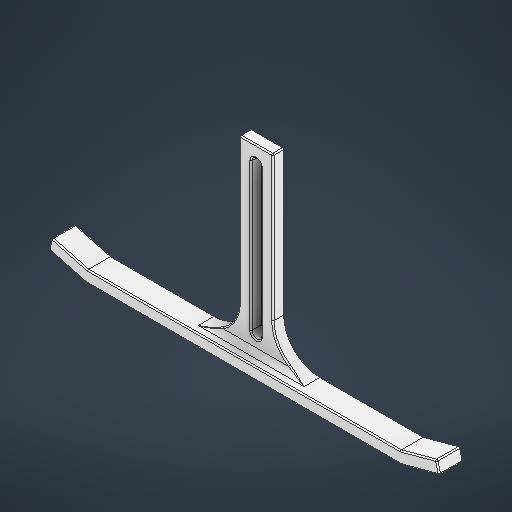
# Autodesk Inventor part: BandeV2Joint3_HALF
Saved by Autodesk Inventor 2026.2 (Build 302298010, 298A)
## iProperties
Created: 2026-06-25
Part Number: BandeV2Joint3_HALF
Material: PET Plastic
Document SubType Name: Modeling
Designer: frede
Density: 1.541 g/cm^3
Appearance: White
Author: frede
Autodesk Inventor part; units mm, degrees
ref_plane "YZ Plane" through (0, 0, 0) normal (1, 0, 0) x (0, 1, 0)
ref_plane "XZ Plane" through (0, 0, 0) normal (0, 1, 0) x (-1, 0, 0)
ref_plane "XY Plane" through (0, 0, 0) normal (0, 0, 1) x (1, 0, 0)
sketch "Sketch1" plane through (0, 0, 0) normal (0, 0, 1) x (1, 0, 0)
  line L0 (0, 0) -> (14, 0)
  line L1 (14, 0) -> (14, -75)
  line L2 (14, -75) -> (0, -75)
  line L3 (0, -75) -> (0, 0)
  arc A0 (4.875, -68) -> (9.125, -68) centre (7, -68) ccw
  arc A1 (9.125, -7) -> (4.875, -7) centre (7, -7) ccw
  line L4 (9.125, -7) -> (9.125, -68)
  line L5 (4.875, -68) -> (4.875, -7)
  line L6 (0, -75) -> (-58, -75)
  line L7 (-58, -75) -> (-73, -70.9808)
  line L8 (14, -75) -> (72, -75)
  line L9 (72, -75) -> (87, -70.9808)
  line L10 (88.2941, -75.8104) -> (72.6583, -80)
  line L11 (-74.2941, -75.8104) -> (-58.6583, -80)
  line L12 (72.6583, -80) -> (-58.6583, -80)
  line L13 (87, -70.9808) -> (88.2941, -75.8104)
  line L14 (-73, -70.9808) -> (-74.2941, -75.8104)
  point P0 (7, -75)
  dimension "d0" = 75
  dimension "d1" = 14
  dimension "d2" = 4.25
  dimension "d3" = 4.25
  dimension "d4" = 7
  dimension "d5" = 7
  dimension "d7" = 165
  dimension "d9" = 165
  dimension "d10" = 160
  dimension "d11" = 15
  dimension "d12" = 15
  dimension "d13" = 80
  dimension "d14" = 4.875
  dimension "d15" = 5
  dimension "d16" = 5
  dimension "d17" = 5
  constraints: 30 end point, 5 parallel, 4 horizontal, 4 point on circle, 3 perpendicular, 3 tangent, 2 centre point, 1 midpoint
  measures "d0" distance between parallel lines of L0 L2
  measures "d1" distance between parallel lines of L3 L1
  measures "d2" diameter of A0
  measures "d3" diameter of A1
  measures "d4" distance from line of L2 A0.centre
  measures "d5" distance from line of L0 A1.centre
  measures "d7" angle of L6 L7
  measures "d9" angle of L9 L8
  measures "d10" distance of L7.end L9.end
  measures "d11" horizontal distance of L8.end L9.end
  measures "d12" horizontal distance of L7.end L6.end
  measures "d13" horizontal distance of L7.end point (7, -75)
  measures "d14" distance between parallel lines of L3 L5
  measures "d15" distance between parallel lines of L7 L11
  measures "d16" distance between parallel lines of L9 L10
  measures "d17" distance between parallel lines of L8 L12
extrude "Extrusion1" add sketch "Sketch1" along normal blind 5 contours L0 L1 L2 L3
extrude "Extrusion2" add sketch "Sketch1" along normal blind 10 contours L2 L8 L9 L13 L10 L12 L11 L14 L7 L6
fillet "Fillet1" radius 15 2 edges at (0, -75, 2.5) (14, -75, 2.5)
fillet "Fillet2" radius 2 3 edges at (-7.5, -75, 5) (7, -75, 5) (21.5, -75, 5)
fillet "Fillet3" radius 0.5 43 edges at (7, 0, 5) (16.0144, -67.5083, 5) (25.2504, -74.5238, 5.7046) (14, -30, 5) (18.3934, -70.6066, 0) (50.5, -75, 0) (14, -30, 0) (7, -4.875, 5) (9.125, -37.5, 5) (7, -70.125, 5) (4.875, -37.5, 5) (-2.0144, -67.5083, 5) (-11.2504, -74.5238, 5.7046) (0, -30, 5) (-4.3934, -70.6066, 0) (-36.5, -75, 0) (0, -30, 0) (7, -4.875, 0) (9.125, -37.5, 0) (7, -70.125, 0) (4.875, -37.5, 0) (7, 0, 0) (0, 0, 2.5) (14, 0, 2.5) (7, -75, 10) (79.5, -72.9904, 10) (87, -70.9808, 5) (79.5, -72.9904, 0) (88.2941, -75.8104, 5) (87.647, -73.3956, 10) (80.4762, -77.9052, 10) (87.647, -73.3956, 0) (80.4762, -77.9052, 0) (7, -80, 10) (7, -80, 0) (-66.4762, -77.9052, 10) (-65.5, -72.9904, 10) (-73.647, -73.3956, 10) (-65.5, -72.9904, 0) (-73.647, -73.3956, 0) (-73, -70.9808, 5) (-74.2941, -75.8104, 5) (-66.4762, -77.9052, 0)
equation "\"d13\" = 0.5 * d10"
equation "\"d14\" = -0.5 * d2 + 0.5 * d1"
equation "\"d15\" = d17"
equation "\"d16\" = d17"
body "Solid1"
